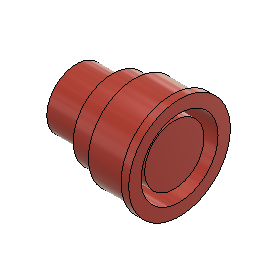
DIN 5 connector (Autodesk Fusion 360 design; units mm, degrees)
Autodesk Fusion 360 part; units mm, degrees
sketch "DIN 5 connector" plane through (0, 0, 0) normal (0, 0, 1) x (1, 0, 0)
  circle A0 centre (0, 0) radius 9.85
  circle A1 centre (0, 0) radius 7.625
  circle A2 centre (0, 0) radius 5.75
  circle A3 centre (0, 0) radius 8.975
  circle A4 centre (0, 0) radius 7.475
  dimension "d58" = 19.7
  dimension "d59" = 15.25
  dimension "d60" = 11.5
  dimension "d61" = 17.95
  dimension "d62" = 14.95
  dimension "d156" = 0
  dimension "d157" = 0
  dimension "d158" = 0
  dimension "d159" = 0
  dimension "d168" = 0
  dimension "d169" = 0
  dimension "d170" = 0
  dimension "d171" = 0
  constraint coincident A0.centre A1.centre
  constraint concentric A0 A3
  constraint concentric A0 A4
  measures "d58" diameter of A0
  measures "d59" diameter of A1
  measures "d60" diameter of A2
  measures "d61" diameter of A3
  measures "d62" diameter of A4
extrude "Extrude1" add sketch "DIN 5 connector" along normal blind 1.5 contours A0 | A1 | A2 | A3 | A4
extrude "Extrude2" add sketch "DIN 5 connector" along normal blind 8.7 contours A1 | A2 | A3 | A4
extrude "Extrude3" add sketch "DIN 5 connector" along normal blind 13 contours A1 | A2 | A4
extrude "Extrude4" add sketch "DIN 5 connector" along normal blind 20 contours A2
extrude "Extrude5" cut sketch "DIN 5 connector" along normal blind 7 contours A4
extrude "Extrude6" cut sketch "DIN 5 connector" along normal blind 1 contours A2
move_body "Move1" bodies 1 to x (0, 0, -1) y (0, 1, 0) z (1, 0, 0) at (-9.85, 0, -9.85)
move_body "Move2" bodies 1 to x (-1, 0, 0) y (0, 1, 0) z (0, 0, -1) at (-19.7, 0, -39.4)
named bodies: "DIN 5 connector"
